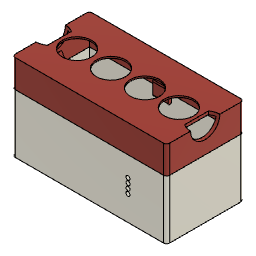
block-four-fingerjoysticks v8 (Autodesk Fusion 360 design; units mm, degrees)
Autodesk Fusion 360 part; units mm, degrees
note: some values were not read from the file. Set by a fixed rule: which face or edge a step refers to.
sketch "bottom" plane through (0, 0, 0) normal (0, 0, 1) x (1, 0, 0) in component "bottom"
  line L0 (50, 25) -> (-50, 25)
  line L1 (-50, 25) -> (-50, -25)
  line L2 (-50, -25) -> (50, -25)
  line L3 (50, -25) -> (50, 25)
  line L4 (50, 25) -> (-50, -25) construction
  line L5 (-50, 25) -> (50, -25) construction
  dimension "d5" = 100
  dimension "d6" = 50
  constraint perpendicular L0 L1
  constraint parallel L0 L2
  constraint parallel L1 L3
  constraint horizontal L0
  constraint coincident L4 origin
  constraint coincident L5 origin
  measures "d5" distance of L1.end L2.end
  measures "d6" distance of L0.end L1.end
extrude "Extrude1" add sketch "bottom" along normal blind 38 makes body 1 in component "bottom"
fillet "Fillet1" radius 2 4 edges at (50, 25, 19) (-50, 25, 19) (-50, -25, 19) (50, -25, 19) on bodies 1 in component "bottom"
shell "Shell1" thickness 2 removed faces 1 at (-16, -8.3333, 38) on bodies 1 in component "bottom"
ref_plane "WorkPlane1" through (0, 0, 56) normal (0, 0, 1) x (1, 0, 0) in component "top"
sketch "top" plane through (0, 0, 56) normal (0, 0, 1) x (1, 0, 0) in component "top"
  line L0 (50, -25) -> (-50, -25)
  line L1 (-50, -25) -> (-50, 25)
  line L2 (-50, 25) -> (50, 25)
  line L3 (50, 25) -> (50, -25)
  line L4 (50, -25) -> (-50, 25) construction
  line L5 (-50, -25) -> (50, 25) construction
  dimension "d12" = 50
  dimension "d13" = 100
  constraint perpendicular L0 L1
  constraint parallel L0 L2
  constraint parallel L1 L3
  constraint horizontal L0
  constraint coincident L4 origin
  constraint coincident L5 origin
  measures "d12" distance of L0.end L1.end
  measures "d13" distance of L1.end L2.end
extrude "Extrude1'" add sketch "top" against normal blind 18 separate body makes body 2 in component "top"
fillet "Fillet1'" radius 2 4 edges at (-50, 25, 47) (50, 25, 47) (50, -25, 47) (-50, -25, 47) on bodies 2 in component "top"
shell "Shell1'" thickness 2 removed faces 1 at (-16, 8.3333, 38) on bodies 2 in component "top"
sketch "holes" plane through (0, 0, 2) normal (0, 0, 1) x (1, 0, 0) in component "bottom"
  line L0 (48, 23) -> (-48, 23)
  line L1 (-48, 23) -> (-48, -23)
  line L2 (-48, -23) -> (48, -23)
  line L3 (48, -23) -> (48, 23)
  line L4 (25, 31.2139) -> (25, -33.1934) construction
  line L5 (-48, 23) -> (48, 23)
  line L6 (48, 23) -> (48, -23)
  line L7 (48, -23) -> (-48, -23)
  line L8 (-48, -23) -> (-48, 23)
  arc A0 (48, -25) -> (50, -23) centre (48, -23) ccw
  line L9 (50, -23) -> (50, 23)
  arc A1 (50, 23) -> (48, 25) centre (48, 23) ccw
  line L10 (48, 25) -> (-48, 25)
  arc A2 (-48, 25) -> (-50, 23) centre (-48, 23) ccw
  line L11 (-50, 23) -> (-50, -23)
  arc A3 (-50, -23) -> (-48, -25) centre (-48, -23) ccw
  line L12 (-48, -25) -> (48, -25)
  line L13 (0, 2.5) -> (0, 20)
  circle A4 centre (36, 11) radius 6.25
  circle A5 centre (36, -11) radius 6.25
  circle A6 centre (14, 11) radius 6.25
  circle A7 centre (14, -11) radius 6.25
  circle A8 centre (25, -5) radius 1.3
  circle A9 centre (25, -8) radius 1.3
  circle A10 centre (25, -11) radius 1.3
  circle A11 centre (25, -14) radius 1.3
  line L14 (25, -5) -> (25, 0)
  line L15 (28, -3) -> (22, -3)
  line L16 (22, -3) -> (22, 3)
  line L17 (22, 3) -> (28, 3)
  line L18 (28, 3) -> (28, -3)
  line L19 (28, -3) -> (22, 3) construction
  line L20 (22, -3) -> (28, 3) construction
  point P0 (36, -11)
  point P1 (25, -14)
  point P2 (25, -11)
  point P3 (25, -8)
  point P4 (25, -5)
  point P5 (36, 11)
  point P6 (14, 11)
  point P7 (14, -11)
  point P8 (25, 0)
  dimension "d90" = 0
  dimension "distancePins" = 3
  dimension "d114" = 25
  dimension "marginPins" = 11
  dimension "d116" = 14
  dimension "d117" = 11
  dimension "d118" = 22
  dimension "d167" = 12.5
  dimension "d168" = 12.5
  dimension "d169" = 12.5
  dimension "d170" = 12.5
  dimension "d171" = 2.6
  dimension "d172" = 2.6
  dimension "d173" = 2.6
  dimension "d174" = 2.6
  dimension "d200" = 5
  dimension "d201" = 6
  dimension "d202" = 6
  constraint vertical L4
  constraint coincident P1 L4
  constraint vertical P0 A4.centre
  constraint symmetric P0 L4 P7
  constraint symmetric L4 P5 P6
  constraint coincident P5 A4.centre
  constraint coincident P0 A5.centre
  constraint coincident P6 A6.centre
  constraint coincident P7 A7.centre
  constraint coincident P4 A8.centre
  constraint coincident P3 A9.centre
  constraint coincident P2 A10.centre
  constraint coincident P1 A11.centre
  constraint parallel L4 L14
  constraint perpendicular L15 L16
  constraint parallel L15 L17
  constraint parallel L16 L18
  constraint horizontal L15
  constraint coincident L19 P8
  constraint coincident L20 P8
  constraint coincident P8 L14.end
  measures "d114" distance of L4 L9
  measures "marginPins" distance of P1 L12
  measures "d116" distance of P0 L12
  measures "d117" distance of P0 L4
  measures "d118" distance of P0 A4.centre
  measures "d167" diameter of A4
  measures "d168" diameter of A5
  measures "d169" diameter of A6
  measures "d170" diameter of A7
  measures "d171" diameter of A8
  measures "d172" diameter of A9
  measures "d173" diameter of A10
  measures "d174" diameter of A11
  measures "d200" distance of P4 P8
  measures "d201" distance of L16.end L17.end
  measures "d202" distance of L15.end L16.end
extrude "Extrude6" cut sketch "holes" against normal blind 1 contours A4 | A5 | A6 | A7 bodies 1 in component "bottom"
extrude "Extrude7" cut sketch "holes" against normal blind 2 contours A8 | A9 | A10 | A11 bodies 1 in component "bottom"
sketch "handle" plane through (50, 0, 0) normal (1, 0, 0) x (0, 0, -1) in component "top"
  line L0 (-38, -23) -> (-38, 23)
  line L1 (-56, 23) -> (-56, -23)
  line L2 (-56, 23) -> (-56, -23)
  circle A0 centre (-56, 0) radius 7.5
  line L3 (-56, -23) -> (-38, -23)
  line L4 (-38, 23) -> (-56, 23)
  line L5 (-38, 23) -> (-38, -23)
  circle A1 centre (-56, 0) radius 9.5
  dimension "d95" = 15
  dimension "d159" = 2
  constraint midpoint L1 A0.centre
  constraint concentric A0 A1
  measures "d95" diameter of A0
  measures "d159" distance of A0 A1
revolve "Revolve1" cut sketch "handle" angle 90 about axis through (50, 23, 56) along (0, 1, 0) contours L1 L2 A0 picked at (-53.2397, 2.1031) bodies 2 in component "top"
revolve "Revolve2" cut sketch "handle" angle 90 about axis through (50, 23, 56) along (0, 1, 0) contours L1 L2 A0 A1 picked at (-55.1935, 8.7757) bodies 2 in component "top"
mirror "Mirror9" about plane through (0, 0, 0) normal (1, 0, 0) of "Revolve1", "Revolve2" in component "top"
sketch "customisable" plane through (0, 0, 56) normal (0, 0, 1) x (1, 0, 0) in component "top"
  line L0 (-50, -9.5) -> (-50, -23)
  line L1 (-48, -25) -> (48, -25)
  line L2 (48, 25) -> (-48, 25)
  line L3 (0.05, 0.05) -> (-0.05, 0.05)
  line L4 (-0.05, 0.05) -> (-0.05, -0.05)
  line L5 (-0.05, -0.05) -> (0.05, -0.05)
  line L6 (0.05, -0.05) -> (0.05, 0.05)
  line L7 (0.05, 0.05) -> (-0.05, -0.05) construction
  line L8 (-0.05, 0.05) -> (0.05, -0.05) construction
  arc A0 (-50, -23) -> (-48, -25) centre (-48, -23) ccw
  arc A1 (48, -25) -> (50, -23) centre (48, -23) ccw
  line L9 (50, -23) -> (50, -9.5)
  arc A2 (50, 23) -> (48, 25) centre (48, 23) ccw
  arc A3 (-48, 25) -> (-50, 23) centre (-48, 23) ccw
  arc A4 (-50, -9.5) -> (-50, 9.5) centre (-50, 0) ccw
  arc A5 (50, 9.5) -> (50, -9.5) centre (50, 0) ccw
  line L10 (50, 9.5) -> (50, 23)
  line L11 (-50, 23) -> (-50, 9.5)
  dimension "d104" = 0.1
  dimension "d105" = 0.1
  constraint perpendicular L3 L4
  constraint parallel L3 L5
  constraint parallel L4 L6
  constraint horizontal L3
  constraint coincident L7 origin
  constraint coincident L8 origin
  measures "d104" distance of L3.start L3.end
  measures "d105" distance of L3.start L5.end
extrude "Extrude4" [suppressed] in component "top"
extrude "Extrude8" cut sketch "holes" against normal blind 1 contours L15 L16 L17 L18 bodies 1 in component "bottom"
pattern_linear "R-Pattern1" count 1 spacing 50 along (0, 1, 0) count 2 spacing 50 along (-1, 0, 0) of "Extrude6" in component "bottom"
sketch "snap" plane through (0, 0, 0) normal (1, 0, 0) x (0, 0, -1) in component "top"
  line L0 (-28, -48) -> (0, -48)
  line L1 (0, -48) -> (0, 48)
  line L2 (0, 48) -> (-28, 48)
  line L3 (-28, 48) -> (-28, -48)
  arc A0 (-38, 23) -> (-37.2488, 23.2186) centre (-38, 24.4) ccw
  line L4 (-37.2488, 23.2186) -> (-36.3595, 23.7321)
  arc A1 (-34.3595, 23.7321) -> (-36.3595, 23.7321) centre (-35.3595, 22) ccw
  line L5 (-34.3595, 23.7321) -> (-33.0915, 23)
  arc A2 (-32.5957, 22.2256) -> (-33.0915, 23) centre (-33.5915, 22.134) ccw
  line L6 (-32.5957, 22.2256) -> (-32.5834, 22.0917)
  arc A3 (-33.5792, 21) -> (-32.5834, 22.0917) centre (-33.5792, 22) ccw
  line L7 (-33.5792, 21) -> (-40.9732, 21)
  arc A4 (-42.0232, 21.2813) -> (-40.9732, 21) centre (-40.9732, 23.1) ccw
  line L8 (-42.0232, 21.2813) -> (-45, 23)
  line L9 (-45, 23) -> (-38, 23)
  line L10 (-54, 23) -> (-38, 23)
  line L11 (-38, 23) -> (-54, 23)
  dimension "d140" = 2
  dimension "d141" = 1
  dimension "d143" = 2.1
  dimension "d144" = 1.4
  dimension "d145" = 2
  dimension "d146" = 30
  dimension "d147" = 150
  dimension "d148" = 30
  dimension "d149" = 1
  dimension "d150" = 7
  constraint tangent A0 L9
  constraint horizontal L9
  constraint horizontal L7
  constraint tangent L4 A1
  constraint tangent A1 L5
  constraint tangent L5 A2
  constraint tangent A3 L7
  constraint tangent L7 A4
  constraint tangent A4 L8
  constraint tangent A2 L6
  constraint tangent L6 A3
  constraint horizontal A0.start L5.end
  constraint equal A2 A3
  constraint coincident A0.start L9.end
  measures "d140" radius of A1
  measures "d141" radius of A2
  measures "d143" radius of A4
  measures "d144" radius of A0
  measures "d145" distance of A0.start L7
  measures "d146" angle of L8 L9
  measures "d147" angle of L4 L9
  measures "d148" angle of L5 L9
  measures "d149" vertical distance of A0.start A1.centre
  measures "d150" distance of A0.start L8.end
extrude "Extrude5" add sketch "snap" along normal mid plane 10 separate body contours A0 L4 A1 L5 A2 L6 A3 L7 A4 L8 L9 L10 L11 makes body 3 in component "top"
mirror "Mirror6" about plane through (0, 0, 0) normal (0, 1, 0) of "Extrude5" makes body 4 in component "top"
copy_body "CopyPasteBodies2" bodies 3 makes body 5 in component "top"
move_body "Move4" bodies 5 to x (0, -1, 0) y (1, 0, 0) z (0, 0, 1) at (-26, 16, 0) in component "top"
move_body "Move5" bodies 5 to x (1, 0, 0) y (0, 1, 0) z (0, 0, 1) at (51, -16, 0) in component "top"
mirror "Mirror7" about plane through (0, 0, 0) normal (1, 0, 0) of bodies 5 makes body 6 in component "top"
combine "Combine1" operation cut target body 1 tool bodies 3 6 4 5 keep tools in component "bottom"
move_face "OffsetFaces1" offset -0.1 24 faces at (1.6667, -23.0062, 37.868) (-1.6667, -23.3898, 36.9523) (1.6667, -23.7797, 36.2719) (-1.6667, -23.488, 33.9368) (-5, -23.3169, 34.8999) (5, -23.3169, 34.8999) (-48.7797, -1.6667, 36.2719) (-48.3898, 1.6667, 36.9523) (-48.1845, 1.6667, 37.3053) (-48.488, 1.6667, 33.9368) (-48.3169, -5, 34.8999) (-48.3169, 5, 34.8999) (1.6667, 23.0062, 37.868) (-1.6667, 23.3898, 36.9523) (1.6667, 23.7797, 36.2719) (-1.6667, 23.488, 33.9368) (5, 23.3169, 34.8999) (-5, 23.3169, 34.8999) (48.3169, 5, 34.8999) (48.7797, -1.6667, 36.2719) (48.488, 1.6667, 33.9368) (48.3898, 1.6667, 36.9523) (48.1845, 1.6667, 37.3053) (48.3169, -5, 34.8999) on bodies 1 in component "bottom"
combine "Combine2" operation add target body 2 tool bodies 3 4 6 5 in component "top"
ref_plane "WorkPlane1" through (0, -25, 47) normal (0, -1, 0) x (-1, 0, 0)
sketch "sideHoles" plane through (0, -25, 11) normal (0, -1, 0) x (1, 0, 0)
  circle A0 centre (0, 17) radius 1
  arc A1 (-23, 25) -> (-25, 23) centre (-23, 23) ccw
  line L0 (19.7878, 45) -> (19.7878, 25)
  arc A2 (-25, -23) -> (-23, -25) centre (-23, -23) ccw
  arc A3 (25, 23) -> (23, 25) centre (23, 23) ccw
  line L1 (-25, 23) -> (-25, -23)
  line L2 (23, 25) -> (-23, 25)
  circle A4 centre (0, 14) radius 1
  circle A5 centre (0, 8) radius 1
  line L3 (25, -23) -> (25, 23)
  arc A6 (23, -25) -> (25, -23) centre (23, -23) ccw
  circle A7 centre (0, 11) radius 1
  line L4 (-23, -25) -> (23, -25)
  line L5 (19.7878, 25) -> (-20.2122, 25)
  line L6 (-20.2122, 45) -> (19.7878, 45)
  line L7 (-20.2122, 25) -> (-20.2122, 45)
sketch "holesWithMagnets" plane through (0, -23, 0) normal (0, 1, 0) x (1, 0, 0) in component "bottom"
  line L0 (0, -34) -> (0, 12) construction
  circle A0 centre (36, -22) radius 6.25
  line L1 (0, -8.617) -> (0, 8.883)
  arc A1 (2, -36) -> (0, -34) centre (2, -34) cw construction
  arc A2 (0, 12) -> (2, 14) centre (2, 12) cw construction
  arc A3 (48, 14) -> (50, 12) centre (48, 12) cw construction
  circle A4 centre (25, -19) radius 1.3
  line L2 (50, 12) -> (50, -34) construction
  circle A5 centre (36, 0) radius 6.25
  arc A6 (50, -34) -> (48, -36) centre (48, -34) cw construction
  circle A7 centre (14, -22) radius 6.25
  line L3 (2, 14) -> (48, 14) construction
  circle A8 centre (14, 0) radius 6.25
  circle A9 centre (25, -16) radius 1.3
  line L4 (48, -36) -> (2, -36) construction
  circle A10 centre (25, -22) radius 1.3
  circle A11 centre (25, -25) radius 1.3
  line L5 (5.1, -38) -> (48, -38)
  line L6 (48, -38) -> (48, -2)
  line L7 (48, -2) -> (-48, -2)
  line L8 (-48, -2) -> (-48, -38)
  line L9 (25, -16) -> (25, -11) construction
  line L10 (22, -8) -> (28, -8)
  line L11 (28, -8) -> (28, -14)
  line L12 (28, -14) -> (22, -14)
  line L13 (22, -14) -> (22, -8)
  line L14 (22, -8) -> (28, -14) construction
  line L15 (28, -8) -> (22, -14) construction
  line L16 (36, -22) -> (36, 0) construction
  line L17 (36, 0) -> (14, 0) construction
  line L18 (14, 0) -> (14, -22) construction
  line L19 (14, -22) -> (36, -22) construction
  line L20 (25, -16) -> (25, -19) construction
  line L21 (25, -19) -> (25, -22) construction
  line L22 (25, -25) -> (25, -22) construction
  line L23 (25, -19) -> (25, -16) construction
  line L24 (25, -19) -> (25, -22) construction
  line L25 (50, 0) -> (50, -38)
  line L26 (48, -56) -> (-48, -56)
  line L27 (5.1, -32.8915) -> (5.1, -38)
  line L28 (-48, -38) -> (-5.1, -38)
  line L29 (-5.1, -38) -> (-5.1, -32.8915)
  line L30 (-5.1, -32.8915) -> (5.1, -32.8915)
  point P0 (25, -11)
  dimension "d181" = 5
  dimension "d182" = 6
  dimension "d183" = 6
  dimension "d190" = 3
  dimension "d191" = 3
  dimension "d192" = 22
  dimension "d193" = 22
  dimension "d194" = 22
  dimension "d195" = 3
  dimension "d196" = 22
  dimension "d197" = 14
  dimension "d198" = 14
  dimension "d199" = 20
  dimension "d209" = 2.6
  dimension "d211" = 2.6
  dimension "d212" = 2.6
  dimension "d213" = 2.6
  constraint perpendicular L10 L11
  constraint parallel L10 L12
  constraint parallel L11 L13
  constraint horizontal L10
  constraint coincident L14 P0
  constraint coincident L15 P0
  constraint coincident P0 L9.end
  constraint coincident A9.centre L9.start
  constraint coincident A0.centre L16.start
  constraint coincident A5.centre L16.end
  constraint perpendicular L7 L16
  constraint coincident A8.centre L17.end
  constraint perpendicular L16 L17
  constraint coincident A7.centre L18.end
  constraint coincident A4.centre L20.end
  constraint parallel L9 L20
  constraint coincident A10.centre L21.end
  constraint perpendicular L19 L21
  constraint coincident A11.centre L22.start
  constraint perpendicular L19 L22
  constraint collinear L2 L25
  measures "d181" distance of A9.centre P0
  measures "d182" distance of L10.end L11.end
  measures "d183" distance of L11.end L12.end
  measures "d190" distance of A4.centre A10.centre
  measures "d191" distance of A10.centre A11.centre
  measures "d192" distance of A0.centre A7.centre
  measures "d193" distance of A7.centre A8.centre
  measures "d194" distance of A5.centre A8.centre
  measures "d195" distance of A4.centre A9.centre
  measures "d196" distance of A0.centre A5.centre
  measures "d197" distance of L4 A0.centre
  measures "d198" distance of L2 A0.centre
  measures "d199" distance of L4 L26
  measures "d209" diameter of A11
  measures "d211" diameter of A10
  measures "d212" diameter of A4
  measures "d213" diameter of A9
extrude "Extrude4'" cut sketch "holesWithMagnets" against normal blind 1 contours A0 | A7 bodies 1 in component "bottom"
extrude "Extrude11" cut sketch "holesWithMagnets" against normal blind 1 contours L10 L11 L12 L13 bodies 1 in component "bottom"
extrude "Extrude5'" cut sketch "holesWithMagnets" against normal blind 2 contours A4 | A9 | A10 | A11 bodies 1 in component "bottom"
sketch "skirt" plane through (0, 0, 2) normal (0, 0, 1) x (1, 0, 0) in component "bottom"
  line L0 (22, -3) -> (22, 3)
  line L1 (22, 3) -> (28, 3)
  line L2 (28, 3) -> (28, -3)
  line L3 (28, -3) -> (22, -3)
  circle A0 centre (25, -8) radius 1.3
  circle A1 centre (25, -11) radius 1.3
  circle A2 centre (25, -5) radius 1.3
  circle A3 centre (25, -14) radius 1.3
  circle A4 centre (14, 11) radius 6.25
  circle A5 centre (36, -11) radius 6.25
  circle A6 centre (36, 11) radius 6.25
  circle A7 centre (14, -11) radius 6.25
  line L4 (48, 23) -> (-48, 23)
  line L5 (-48, 23) -> (-48, -23)
  line L6 (-48, -23) -> (48, -23)
  line L7 (48, -23) -> (48, 23)
  line L8 (20.7094, 5.0189) -> (29.4652, 5.0189)
  line L9 (22, -15.9265) -> (22, 3)
  line L10 (29.4652, -18.542) -> (20.7094, -18.542)
  line L11 (28.0623, -15.9265) -> (22, -15.9265)
  line L12 (29.4652, 5.0189) -> (29.4652, -18.542)
  line L13 (22, 3) -> (28.0623, 3)
  line L14 (28.0623, 3) -> (28.0623, -15.9265)
  line L15 (20.7094, -18.542) -> (20.7094, 5.0189)
  line L16 (20.7094, 5.0189) -> (22, 5.0189)
  line L17 (22, 5.0189) -> (22, 3)
  line L18 (22, 3) -> (20.7094, 3)
  line L19 (20.7094, 3) -> (20.7094, 5.0189)
  line L20 (28.0623, -15.9265) -> (29.4652, -15.9265)
  line L21 (29.4652, -15.9265) -> (29.4652, -18.542)
  line L22 (29.4652, -18.542) -> (28.0623, -18.542)
  line L23 (28.0623, -18.542) -> (28.0623, -15.9265)
  circle A8 centre (-36, 11) radius 6.25
  circle A9 centre (-14, -11) radius 6.25
  circle A10 centre (-14, 11) radius 6.25
  circle A11 centre (-36, -11) radius 6.25
  constraint horizontal L16
  constraint vertical L17
  constraint horizontal L18
  constraint vertical L19
  constraint horizontal L20
  constraint vertical L21
  constraint horizontal L22
  constraint vertical L23
  constraint coincident L0.end L1.start
extrude "Extrude9" add sketch "skirt" along normal blind 0.85 contours L0 L9 L10 L11 L15 L18 L23 | L1 L8 L12 L13 L14 L17 L20 | L8 L15 L16 L17 L18 L19 | L10 L12 L20 L21 L22 L23 bodies 1 in component "bottom"
sketch "skirt_side" plane through (0, -23, 0) normal (0, 1, 0) x (-1, 0, 0) in component "bottom"
  circle A0 centre (-25, 19) radius 1.3
  circle A1 centre (-25, 22) radius 1.3
  circle A2 centre (-25, 16) radius 1.3
  circle A3 centre (-25, 25) radius 1.3
  circle A4 centre (-14, 22) radius 6.25
  circle A5 centre (-36, 22) radius 6.25
  line L0 (-5.1, 32.8915) -> (-5.1, 38)
  line L1 (-5.1, 38) -> (-48, 38)
  line L2 (-48, 38) -> (-48, 2)
  line L3 (-48, 2) -> (48, 2)
  line L4 (48, 2) -> (48, 38)
  line L5 (48, 38) -> (5.1, 38)
  line L6 (5.1, 38) -> (5.1, 32.8915)
  line L7 (5.1, 32.8915) -> (-5.1, 32.8915)
  line L8 (-22, 8) -> (-28, 8)
  line L9 (-28, 8) -> (-28, 26.6255)
  line L10 (-28, 26.6255) -> (-22, 26.6255)
  line L11 (-22, 26.6255) -> (-22, 8)
  line L12 (-20.6516, 5.45) -> (-29.3992, 5.45)
  line L13 (-29.3992, 5.45) -> (-29.3992, 29.1755)
  line L14 (-29.3992, 29.1755) -> (-20.6516, 29.1755)
  line L15 (-20.6516, 29.1755) -> (-20.6516, 5.45)
  line L16 (-28, 8) -> (-28, 14)
  line L17 (-28, 14) -> (-22, 14)
  line L18 (-22, 14) -> (-22, 8)
  line L19 (-22, 8) -> (-28, 8)
  line L20 (-20.6516, 5.45) -> (-22, 5.45)
  line L21 (-22, 5.45) -> (-22, 8)
  line L22 (-22, 8) -> (-20.6516, 8)
  line L23 (-20.6516, 8) -> (-20.6516, 5.45)
  line L24 (-28, 26.6255) -> (-29.3992, 26.6255)
  line L25 (-29.3992, 26.6255) -> (-29.3992, 29.1755)
  line L26 (-29.3992, 29.1755) -> (-28, 29.1755)
  line L27 (-28, 29.1755) -> (-28, 26.6255)
  dimension "d216" = 2.55
  dimension "d217" = 2.55
  constraint horizontal L8
  constraint vertical L9
  constraint horizontal L10
  constraint vertical L11
  constraint horizontal L12
  constraint vertical L13
  constraint horizontal L14
  constraint vertical L15
  constraint horizontal L20
  constraint vertical L21
  constraint horizontal L22
  constraint vertical L23
  constraint coincident L8.start L11.end
  constraint horizontal L24
  constraint vertical L25
  constraint horizontal L26
  constraint vertical L27
  measures "d216" distance of L10 L14
  measures "d217" distance of L8 L12
extrude "Extrude10" add sketch "skirt_side" along normal blind 1.1 contours L8 L9 L12 L13 L16 L19 L21 L24 | L12 L15 L20 L21 L22 L23 | L10 L11 L14 L15 L18 L22 L27 | L13 L14 L24 L25 L26 L27 bodies 1 in component "bottom"
chamfer "Chamfer1" distance 1 angle 45 1 edges at (25.0254, -21.9, 5.45) measured on face at (26.0169, -21.9, 6.3) on bodies 1 in component "bottom"
sketch "Sketch3" plane through (0, 0, 2) normal (0, 0, 1) x (1, 0, 0)
  line L0 (48, 23) -> (-48, 23)
  line L1 (-48, 23) -> (-48, -23)
  line L2 (-48, -23) -> (48, -23)
  line L3 (48, -23) -> (48, 23)
  circle A0 centre (14, -11) radius 6.25
  circle A1 centre (36, 11) radius 6.25
  circle A2 centre (36, -11) radius 6.25
  circle A3 centre (14, 11) radius 6.25
  line L4 (-4.3099, -18.4001) -> (-4.3099, 5.1608)
  line L5 (-4.3099, 5.1608) -> (4.4459, 5.1608)
  line L6 (4.4459, 5.1608) -> (4.4459, -18.4001)
  line L7 (4.4459, -18.4001) -> (-4.3099, -18.4001)
  circle A4 centre (-36, -11) radius 6.25
  circle A5 centre (-14, 11) radius 6.25
  circle A6 centre (-14, -11) radius 6.25
  circle A7 centre (-36, 11) radius 6.25
pattern_linear "R-Pattern2" count 2 spacing 50 along (-1, 0, 0) of "Extrude4'" in component "bottom"
sketch "Sketch6" plane through (0, 0, 56) normal (0, 0, 1) x (1, 0, 0) in component "top"
  arc A0 (-50, -9.5) -> (-50, 9.5) centre (-50, 0) ccw
  line L0 (-50, -9.5) -> (-50, -23)
  arc A1 (-50, -23) -> (-48, -25) centre (-48, -23) ccw
  line L1 (-48, -25) -> (48, -25)
  arc A2 (48, -25) -> (50, -23) centre (48, -23) ccw
  line L2 (50, -23) -> (50, -9.5)
  arc A3 (50, 9.5) -> (50, -9.5) centre (50, 0) ccw
  line L3 (50, 9.5) -> (50, 23)
  arc A4 (50, 23) -> (48, 25) centre (48, 23) ccw
  line L4 (48, 25) -> (-48, 25)
  arc A5 (-48, 25) -> (-50, 23) centre (-48, 23) ccw
  line L5 (-50, 23) -> (-50, 9.5)
  line L6 (44.5, 12.5) -> (-44.5, 12.5)
  line L7 (-44.5, 12.5) -> (-44.5, -12.5)
  line L8 (-44.5, -12.5) -> (44.5, -12.5)
  line L9 (44.5, -12.5) -> (44.5, 12.5)
  line L10 (44.5, 12.5) -> (-44.5, -12.5) construction
  line L11 (-44.5, 12.5) -> (44.5, -12.5) construction
  dimension "d236" = 89
  dimension "d237" = 25
  constraint horizontal L6
  constraint perpendicular L6 L7
  constraint parallel L6 L8
  constraint parallel L7 L9
  constraint coincident L10 origin
  constraint coincident L11 origin
  measures "d236" distance of L7.end L8.end
  measures "d237" distance of L6.end L7.end
extrude "Extrude7'" add sketch "Sketch6" against normal blind 2 contours A0 L7 | A0 A3 L6 L7 L8 L9 | A3 L9 bodies 2 in component "top"
sketch "Sketch5" plane through (0, 0, 54) normal (0, 0, -1) x (-1, 0, 0) in component "top"
  arc A0 (44.5, -7.4833) -> (48, -9.0692) centre (50, 0) ccw
  line L0 (48, -23) -> (48, -9.0692)
  line L1 (48, 23) -> (-48, 23)
  line L2 (-48, -9.0692) -> (-48, -23)
  arc A1 (-48, -9.0692) -> (-44.5, -7.4833) centre (-50, 0) ccw
  line L3 (-48, -23) -> (48, -23)
  line L4 (-48, -9.0692) -> (48, -23) construction
  line L5 (48, -9.0692) -> (-48, -23) construction
  line L6 (33, -6) -> (-33, -6) construction
  line L7 (-33, -6) -> (-33, 6) construction
  line L8 (-33, 6) -> (33, 6) construction
  line L9 (33, 6) -> (33, -6) construction
  line L10 (33, -6) -> (-33, 6) construction
  line L11 (-33, -6) -> (33, 6) construction
  circle A2 centre (-33, 0) radius 9.25 construction
  circle A3 centre (-33, 0) radius 9.45
  line L12 (-45.7405, -13.9178) -> (45.7405, -13.9178) construction
  line L13 (45.7405, -13.9178) -> (45.7405, 13.9178) construction
  line L14 (45.7405, 13.9178) -> (-45.7405, 13.9178) construction
  line L15 (-45.7405, 13.9178) -> (-45.7405, -13.9178) construction
  line L16 (-45.7405, -13.9178) -> (45.7405, 13.9178) construction
  line L17 (45.7405, -13.9178) -> (-45.7405, 13.9178) construction
  line L18 (44.5, -7.4833) -> (44.5, 7.4833)
  arc A4 (48, 9.0692) -> (44.5, 7.4833) centre (50, 0) ccw
  line L19 (48, 9.0692) -> (48, 23)
  line L20 (-48, 23) -> (-48, 9.0692)
  arc A5 (-44.5, 7.4833) -> (-48, 9.0692) centre (-50, 0) ccw
  line L21 (-44.5, 7.4833) -> (-44.5, -7.4833)
  circle A6 centre (-33, 0) radius 10.7
  dimension "d230" = 66
  dimension "d231" = 12
  dimension "d232" = 18.5
  dimension "d233" = 0.2
  dimension "d240" = 1.45
  constraint coincident L2.start A1.start
  constraint coincident L0.start L3.end
  constraint coincident A0.end L0.end
  constraint coincident L2.end L3.start
  constraint horizontal L6
  constraint perpendicular L6 L7
  constraint parallel L6 L8
  constraint parallel L7 L9
  constraint coincident L10 origin
  constraint coincident L11 origin
  constraint midpoint L7 A2.centre
  constraint horizontal L12
  constraint perpendicular L12 L13
  constraint parallel L12 L14
  constraint parallel L13 L15
  constraint coincident L16 origin
  constraint coincident L17 origin
  measures "d230" distance of L7.end L8.end
  measures "d231" distance of L6.end L7.end
  measures "d232" diameter of A2
extrude "Extrude8'" cut sketch "Sketch5" against normal blind 2 contours A3 bodies 2 in component "top"
extrude "Extrude9'" cut sketch "Sketch5" against normal blind 1 contours A6 bodies 2 in component "top"
pattern_linear "R-Pattern1'" count 4 spacing 22 along (-1, 0, 0) of "Extrude8'", "Extrude9'" in component "top"
sketch "Sketch7" plane through (0, 0, 54) normal (0, 0, -1) x (-1, 0, 0) in component "top"
  line L0 (43.95, -6) -> (-43.95, -6)
  line L1 (-43.95, -6) -> (-43.95, 6)
  line L2 (-43.95, 6) -> (43.95, 6)
  line L3 (43.95, 6) -> (43.95, -6)
  line L4 (43.95, -6) -> (-43.95, 6) construction
  line L5 (-43.95, -6) -> (43.95, 6) construction
  dimension "d256" = 87.9
  dimension "d257" = 12
  constraint horizontal L0
  constraint perpendicular L0 L1
  constraint parallel L0 L2
  constraint parallel L1 L3
  constraint coincident L4 origin
  constraint coincident L5 origin
  measures "d256" distance of L1.end L2.end
  measures "d257" distance of L0.end L1.end
extrude "Extrude10'" cut sketch "Sketch7" against normal blind 1 bodies 2 in component "top"
component "bottom" placed x (1, 0, 0) y (0, 1, 0) z (0, 0, 1) at (0, 0, 0)
component "top" placed x (1, 0, 0) y (0, 1, 0) z (0, 0, 1) at (0, 0, 0)
equation "height = 56 mm"
equation "d5 = ( width_blocks * 50 ) * 1 mm"
equation "d6 = ( length_blocks * 50 ) * 1 mm"
equation "d7 = height / 2 + 10 mm"
equation "d10 = thickness"
equation "d11 = height"
equation "d12 = ( length_blocks * 50 ) * 1 mm"
equation "d13 = ( width_blocks * 50 ) * 1 mm"
equation "d14 = -height / 2 + 10 mm"
equation "d57 = thickness"
equation "customisable_rectangle = 0.1 mm"
equation "d104 = customisable_rectangle"
equation "d105 = d104"
equation "d119 = length_blocks"
equation "d120 = width_blocks"
equation "width_blocks = 2"
equation "length_blocks = 1"
equation "thickness = 2 mm"
equation "d171 = pinhole"
equation "d172 = pinhole"
equation "d173 = pinhole"
equation "d174 = pinhole"
equation "d175 = -thickness / 2"
equation "d184 = -thickness"
equation "d203 = -thickness / 2"
equation "d205 = -thickness"
equation "d207 = -thickness / 2"
equation "d209 = pinhole"
equation "pinhole = 2.6 mm" comment "Pogo Pin Diameter"
equation "d211 = pinhole"
equation "d212 = pinhole"
equation "d213 = pinhole"
equation "d214 = elevation_bottom_height"
equation "d218 = elevation_side_height"
equation "elevation_bottom_height = 0.85 mm"
equation "elevation_side_height = 1.1 mm"
equation "d224 = width_blocks"
equation "d228 = -thickness / 2"
equation "d230 = spacing * 3"
equation "d232 = diameter"
equation "d233 = tolerance"
equation "d236 = extrusion_handle_correction"
equation "d240 = internal_ring_offset"
equation "d247 = spacing"
equation "spacing = 22 mm"
equation "lateral_margin = 0.8 mm"
equation "diameter = 18.5 mm"
equation "tolerance = 0.2 mm"
equation "internal_ring_offset = tolerance + 1.25 mm"
equation "extrusion_handle_correction = diameter * 4 + ( spacing - diameter ) * 3 + lateral_margin * 2 + internal_ring_offset * 2"
equation "d256 = spacing * 3 + diameter + 2 * internal_ring_offset + 0.5 mm"
named bodies: "bottom", "top", "snap1", "snap2", "snap3", "snap4"
